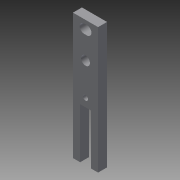
# Autodesk Inventor part: laser supports
Saved by Autodesk Inventor 2013 (Build 170138000, 138)
## iProperties
Created: 2013-07-18
Part Number: laser supports
Material: Generic
Document SubType Name: Modeling
Designer: owner
Density: 1 g/cm^3
Author: owner
Autodesk Inventor part; units mm, degrees
ref_plane "YZ Plane" through (0, 0, 0) normal (1, 0, 0) x (0, 1, 0)
ref_plane "XZ Plane" through (0, 0, 0) normal (0, 1, 0) x (-1, 0, 0)
ref_plane "XY Plane" through (0, 0, 0) normal (0, 0, 1) x (1, 0, 0)
sketch "Sketch1" plane through (0, 0, 0) normal (0, 0, 1) x (1, 0, 0)
  circle A0 centre (0, 330.2) radius 3.175
  arc A1 (0.8308, 346.0532) -> (-0.8308, 346.0532) centre (0, 330.2) ccw
  line L0 (0, 330.2) -> (0.8308, 346.0532) construction
  line L1 (0, 330.2) -> (15.875, 330.2) construction
  line L2 (0, 330.2) -> (-0.8308, 346.0532) construction
  arc A2 (1.1632, 352.3945) -> (-1.1632, 352.3945) centre (0, 330.2) ccw
  arc A3 (-1.1632, 352.3945) -> (-0.8308, 346.0532) centre (-0.997, 349.2239) ccw
  arc A4 (0.8308, 346.0532) -> (1.1632, 352.3945) centre (0.997, 349.2239) ccw
  line L3 (-8.89, 355.1104) -> (-8.89, 265.9564)
  line L4 (-8.89, 355.1104) -> (8.89, 355.1104)
  line L5 (8.89, 355.1104) -> (8.89, 265.9564)
  line L6 (8.89, 265.9564) -> (3.81, 265.9564)
  line L7 (3.81, 265.9564) -> (3.81, 301.5164)
  line L8 (3.81, 301.5164) -> (-3.81, 301.5164)
  line L9 (-3.81, 301.5164) -> (-3.81, 265.9564)
  line L10 (-3.81, 265.9564) -> (-8.89, 265.9564)
  circle A5 centre (0, 307.34) radius 1.778
  point P0 (0, 0)
  dimension "d1" = 6.35
  dimension "d2" = 15.875
  dimension "d3" = 87
  dimension "d4" = 6
  dimension "d7" = 89.154
  dimension "d8" = 17.78
  dimension "d9" = 89.154
  dimension "d10" = 5.08
  dimension "d12" = 35.56
  dimension "d13" = 7.62
  dimension "d15" = 3.556
  constraints: 22 end point, 8 point on circle, 6 centre point, 5 perpendicular, 2 coincident, 2 tangent, 1 equal length, 1 horizontal
  measures "d1" diameter of A0
  measures "d2" radius of A1
  measures "d3" angle of L1 L0
  measures "d4" angle of L0 L2
  measures "d7" distance of L3.start L3.end
  measures "d8" distance of L3.start L4.end
  measures "d9" distance of L4.end L5.end
  measures "d10" distance of L5.end L6.end
  measures "d12" distance of L6.end L7.end
  measures "d13" distance of L7.end L8.end
  measures "d15" diameter of A5
extrude "Extrusion1" add sketch "Sketch1" along normal blind 6.35
body "Solid1"
